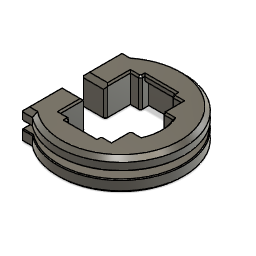
PSUThing (Autodesk Fusion 360 design; units mm, degrees)
Autodesk Fusion 360 part; units mm, degrees
sketch "Skizze1" plane through (0, 0, 0) normal (0, 1, 0) x (1, 0, 0)
  circle A0 centre (0, 0) radius 12.1
  circle A1 centre (0, 0) radius 10.1
  line L0 (0, 0) -> (-40.078, 0) construction
  line L1 (-12.5, 9.6) -> (-12.5, -9.6)
  line L2 (0, 0) -> (20.9765, 0) construction
  line L3 (-12.5, 9.6) -> (-7.3655, 9.6)
  line L4 (-12.5, -9.6) -> (-7.3655, -9.6)
  line L5 (6.5, -10) -> (-6.5, -10)
  line L6 (-6.5, -10) -> (-6.5, 10)
  line L7 (-6.5, 10) -> (6.5, 10)
  line L8 (6.5, 10) -> (6.5, -10)
  line L9 (6.5, -10) -> (-6.5, 10) construction
  line L10 (-6.5, -10) -> (6.5, 10) construction
  line L11 (-3.9, -10) -> (-3.9, 10)
  line L12 (3.9, -10) -> (3.9, 10)
  line L13 (-6.5, -8.9) -> (-3.9, -8.9)
  line L14 (-6.5, 8.9) -> (-3.9, 8.9)
  line L15 (3.9, 8.9) -> (6.5, 8.9)
  line L16 (3.9, -8.9) -> (6.5, -8.9)
  line L17 (6.5, -4) -> (9.2742, -4)
  line L18 (6.5, 4) -> (9.2742, 4)
  point P0 (-12.5, 0)
  point P1 (12.1, 0)
  dimension "d2" = 24.2
  dimension "d3" = 2
  dimension "d4" = 24.6
  dimension "d5" = 19.2
  dimension "d6" = 13
  dimension "d7" = 20
  dimension "d10" = 2.6
  dimension "d11" = 2.6
  dimension "d12" = 1.1
  dimension "d13" = 1.1
  dimension "d14" = 1.1
  dimension "d15" = 1.1
  dimension "d16" = 4
  constraint coincident A0.centre A1.centre
  constraint horizontal L0
  constraint perpendicular L0 L1
  constraint midpoint L1 P0
  constraint coincident L0 P0
  constraint parallel L0 L2
  constraint coincident L2 P1
  constraint coincident A0 P1
  constraint coincident A0 L3.end
  constraint perpendicular L1 L3
  constraint coincident A0 L4.end
  constraint perpendicular L1 L4
  constraint horizontal L5
  constraint perpendicular L5 L6
  constraint parallel L5 L7
  constraint parallel L6 L8
  constraint coincident L9 A0.centre
  constraint coincident L10 A0.centre
  constraint coincident L2 A0.centre
  constraint coincident L5 L11.start
  constraint coincident L7 L11.end
  constraint perpendicular L7 L11
  constraint coincident L5 L12.start
  constraint coincident L7 L12.end
  constraint perpendicular L7 L12
  constraint coincident L6 L13.start
  constraint coincident L11 L13.end
  constraint perpendicular L11 L13
  constraint coincident L6 L14.start
  constraint coincident L11 L14.end
  constraint perpendicular L11 L14
  constraint coincident L12 L15.start
  constraint coincident L8 L15.end
  constraint perpendicular L8 L15
  constraint coincident L12 L16.start
  constraint coincident L8 L16.end
  constraint perpendicular L8 L16
  constraint coincident L8 L17.start
  constraint coincident A1 L17.end
  constraint perpendicular L8 L17
  constraint symmetric L2 L17.start L18.start
  constraint symmetric L2 L17.end L18.end
  measures "d2" diameter of A0
  measures "d3" distance of A0 A1
  measures "d4" distance of P0 P1
  measures "d6" distance of L6.end L7.end
  measures "d7" distance of L5.end L6.end
  measures "d10" distance of L8 L12
  measures "d11" distance of L6 L11
  measures "d12" distance of L5 L16
  measures "d13" distance of L5 L13
  measures "d14" distance of L7 L14
  measures "d15" distance of L7 L15
  measures "d16" distance of L2 L17
extrude "Extrusion1" add sketch "Skizze1" along normal mid plane 1.8 contours A0 | A0 L1 L3 L4 | A1 L8 L18 | A1 L8 L17 | A1 L12 L15 | A1 L7 L8 L12 L15 | A1 L5 L8 L12 L16 | A1 L12 L16 | A1 L7 | A1 L5 | A1 L11 L14 | A1 L6 L7 L11 L14 | A1 L5 L6 L11 L13 | A1 L11 L13 | A1 L6 makes body 1
sketch "Skizze2" plane through (0, -0.9, 0) normal (0, -1, 0) x (1, 0, 0)
  line L0 (3.9, -8.9) -> (3.9, -10)
  line L1 (3.9, -10) -> (-3.9, -10)
  line L2 (-3.9, -10) -> (-3.9, -8.9)
  line L3 (-3.9, -8.9) -> (-6.5, -8.9)
  line L4 (-6.5, -8.9) -> (-6.5, 8.9)
  line L5 (-6.5, 8.9) -> (-3.9, 8.9)
  line L6 (-3.9, 8.9) -> (-3.9, 10)
  line L7 (-3.9, 10) -> (3.9, 10)
  line L8 (3.9, 10) -> (3.9, 8.9)
  line L9 (3.9, 8.9) -> (6.5, 8.9)
  line L10 (6.5, 8.9) -> (6.5, 4)
  line L11 (6.5, 4) -> (9.2742, 4)
  arc A0 (9.2742, -4) -> (9.2742, 4) centre (0, 0) ccw
  line L12 (9.2742, -4) -> (6.5, -4)
  line L13 (6.5, -4) -> (6.5, -8.9)
  line L14 (6.5, -8.9) -> (3.9, -8.9)
  line L15 (-12.5, 9.6) -> (-12.5, -9.6)
  line L16 (-12.5, -9.6) -> (-7.3655, -9.6)
  arc A1 (-7.3655, -9.6) -> (-7.3655, 9.6) centre (0, 0) ccw
  line L17 (-7.3655, 9.6) -> (-12.5, 9.6)
  arc A2 (-9.8003, -12.7736) -> (-9.8003, 12.7736) centre (0, 0) ccw
  line L18 (-12.5, 9.6) -> (-12.5, 17.8119) construction
  line L19 (-12.5, -9.6) -> (-12.5, -17.8838) construction
  line L20 (-9.8003, 12.7736) -> (-12.5, 12.7736)
  line L21 (-12.5, 9.6) -> (-12.5, 12.7736)
  line L22 (-9.8003, -12.7736) -> (-12.5, -12.7736)
  line L23 (-12.5, -12.7736) -> (-12.5, -9.6)
  dimension "d18" = 4
  constraint coincident L15.start L17.end
  constraint perpendicular L17 L18
  constraint coincident L15.end L16.start
  constraint perpendicular L16 L19
  constraint coincident L18 L20.end
  constraint perpendicular L18 L20
  constraint coincident L19 L22.end
  constraint perpendicular L19 L22
extrude "Extrusion2" add sketch "Skizze2" along normal blind 3 bodies 1
sketch "Skizze3" plane through (0, 0.9, 0) normal (0, 1, 0) x (-1, 0, 0)
  line L0 (-3.9, -10) -> (-3.9, -8.9)
  line L1 (-3.9, -8.9) -> (-6.5, -8.9)
  line L2 (-6.5, -8.9) -> (-6.5, -4)
  line L3 (-6.5, -4) -> (-9.2742, -4)
  arc A0 (-9.2742, 4) -> (-9.2742, -4) centre (0, 0) ccw
  line L4 (-9.2742, 4) -> (-6.5, 4)
  line L5 (-6.5, 4) -> (-6.5, 8.9)
  line L6 (-6.5, 8.9) -> (-3.9, 8.9)
  line L7 (-3.9, 8.9) -> (-3.9, 10)
  line L8 (-3.9, 10) -> (3.9, 10)
  line L9 (3.9, 10) -> (3.9, 8.9)
  line L10 (3.9, 8.9) -> (6.5, 8.9)
  line L11 (6.5, 8.9) -> (6.5, -8.9)
  line L12 (6.5, -8.9) -> (3.9, -8.9)
  line L13 (3.9, -8.9) -> (3.9, -10)
  line L14 (3.9, -10) -> (-3.9, -10)
  line L15 (12.5, -9.6) -> (12.5, 9.6)
  line L16 (12.5, 9.6) -> (7.3655, 9.6)
  arc A1 (7.3655, 9.6) -> (7.3655, -9.6) centre (0, 0) ccw
  line L17 (7.3655, -9.6) -> (12.5, -9.6)
  line L18 (12.5, -12.7736) -> (12.5, -9.6)
  line L19 (9.8003, -12.7736) -> (12.5, -12.7736)
  arc A2 (9.8003, 12.7736) -> (9.8003, -12.7736) centre (0, 0) ccw
  line L20 (9.8003, 12.7736) -> (12.5, 12.7736)
  line L21 (12.5, 9.6) -> (12.5, 12.7736)
extrude "Extrusion3" add sketch "Skizze3" along normal blind 3 bodies 1
sketch "Skizze4" plane through (0, 3.9, 0) normal (0, 1, 0) x (-1, 0, 0)
  arc A0 (-9.2742, 4) -> (-9.2742, -4) centre (0, 0) ccw
  line L0 (-9.2742, 4) -> (-6.5, 4)
  line L1 (-6.5, 4) -> (-6.5, 8.9)
  line L2 (-6.5, 8.9) -> (-3.9, 8.9)
  line L3 (-3.9, 8.9) -> (-3.9, 10)
  line L4 (-3.9, 10) -> (3.9, 10)
  line L5 (3.9, 10) -> (3.9, 8.9)
  line L6 (3.9, 8.9) -> (6.5, 8.9)
  line L7 (6.5, 8.9) -> (6.5, -8.9)
  line L8 (6.5, -8.9) -> (3.9, -8.9)
  line L9 (3.9, -8.9) -> (3.9, -10)
  line L10 (3.9, -10) -> (-3.9, -10)
  line L11 (-3.9, -10) -> (-3.9, -8.9)
  line L12 (-3.9, -8.9) -> (-6.5, -8.9)
  line L13 (-6.5, -8.9) -> (-6.5, -4)
  line L14 (-6.5, -4) -> (-9.2742, -4)
  arc A1 (9.8003, 12.7736) -> (9.8003, -12.7736) centre (0, 0) ccw
  line L15 (9.8003, -12.7736) -> (12.5, -12.7736)
  line L16 (12.5, -12.7736) -> (12.5, 12.7736)
  line L17 (12.5, 12.7736) -> (9.8003, 12.7736)
  line L18 (0, 0) -> (25.167, 0) construction
  line L19 (6.5, 0) -> (12.5, 0) construction
  line L20 (6.5, 2.5) -> (12.5, 2.5)
  line L21 (12.5, 2.5) -> (12.5, -2.5)
  line L22 (12.5, -2.5) -> (6.5, -2.5)
  line L23 (6.5, -2.5) -> (6.5, 2.5)
  line L24 (6.5, 2.5) -> (12.5, -2.5) construction
  line L25 (12.5, 2.5) -> (6.5, -2.5) construction
  point P0 (9.5, 0)
  point P1 (9.5, 0)
  dimension "d25" = 5
  constraint coincident A0.centre A1.centre
  constraint perpendicular L16 L18
  constraint midpoint L7 L19.start
  constraint midpoint L16 L19.end
  constraint midpoint L19 P1
  constraint horizontal L20
  constraint perpendicular L20 L21
  constraint parallel L20 L22
  constraint parallel L21 L23
  constraint coincident L7 L20.start
  constraint coincident L24 P1
  constraint coincident L25 P1
  constraint coincident P1 P0
  measures "d25" distance of L20 L22
extrude "Extrusion4" cut sketch "Skizze4" against normal up to surface (7.8 mm away) contours L7 L16 L20 L21 L22 L23 bodies 1
sketch "Skizze5" plane through (0, -3.9, 0) normal (0, -1, 0) x (1, 0, 0)
  line L0 (-6.5, -2.5) -> (-12.5, -2.5)
  line L1 (-12.5, -2.5) -> (-12.5, -12.7736)
  line L2 (-12.5, -12.7736) -> (-9.8003, -12.7736)
  arc A0 (-9.8003, -12.7736) -> (-9.8003, 12.7736) centre (0, 0) ccw
  line L3 (-9.8003, 12.7736) -> (-12.5, 12.7736)
  line L4 (-12.5, 12.7736) -> (-12.5, 2.5)
  line L5 (-12.5, 2.5) -> (-6.5, 2.5)
  line L6 (-6.5, 2.5) -> (-6.5, 8.9)
  line L7 (-6.5, 8.9) -> (-3.9, 8.9)
  line L8 (-3.9, 8.9) -> (-3.9, 10)
  line L9 (-3.9, 10) -> (3.9, 10)
  line L10 (3.9, 10) -> (3.9, 8.9)
  line L11 (3.9, 8.9) -> (6.5, 8.9)
  line L12 (6.5, 8.9) -> (6.5, 4)
  line L13 (6.5, 4) -> (9.2742, 4)
  arc A1 (9.2742, -4) -> (9.2742, 4) centre (0, 0) ccw
  line L14 (9.2742, -4) -> (6.5, -4)
  line L15 (6.5, -4) -> (6.5, -8.9)
  line L16 (6.5, -8.9) -> (3.9, -8.9)
  line L17 (3.9, -8.9) -> (3.9, -10)
  line L18 (3.9, -10) -> (-3.9, -10)
  line L19 (-3.9, -10) -> (-3.9, -8.9)
  line L20 (-3.9, -8.9) -> (-6.5, -8.9)
  line L21 (-6.5, -8.9) -> (-6.5, -2.5)
  line L22 (-3.9, 10) -> (3.9, 10)
  line L23 (3.9, 10) -> (3.9, 11)
  line L24 (3.9, 11) -> (-3.9, 11)
  line L25 (-3.9, 11) -> (-3.9, 10)
  line L26 (0, 0) -> (-17.587, 0) construction
  line L27 (3.9, -11) -> (-3.9, -11)
  line L28 (-3.9, -11) -> (-3.9, -10)
  line L29 (3.9, -10) -> (3.9, -11)
  line L30 (-3.9, -10) -> (3.9, -10)
  dimension "d28" = 1
  constraint perpendicular L22 L23
  constraint parallel L22 L24
  constraint parallel L23 L25
  constraint coincident L9.end L10.start
  constraint perpendicular L10 L22
  constraint coincident L8.end L9.start
  constraint coincident A0.centre A1.centre
  constraint horizontal L26
  constraint symmetric L8.end L26 L18.end
  constraint symmetric L9.end L26 L17.end
  constraint symmetric L23.end L26 L27.start
  constraint symmetric L24.end L26 L27.end
  measures "d28" distance of L8.end L24.end
extrude "Extrusion5" cut sketch "Skizze5" against normal up to surface (6.2 mm away) contours L18 L27 L28 L29 L30 | L9 L22 L23 L24 L25 bodies 1
chamfer "Fase1" distance 1 angle 45 7 edges at (-12.5, 3.9, -7.6368) (-9.5, 3.9, -2.5) (-9.5, 3.9, 2.5) (-12.5, 3.9, 7.6368) (-11.1502, 3.9, 12.7736) (16.1, 3.9, 0) (-11.1502, 3.9, -12.7736) on bodies 1
chamfer "Fase2" distance 0.5 angle 45 8 edges at (-6.5, -0.5, -2.5) (-3.9, 0, -8.9) (3.9, 0, -8.9) (6.5, 0, -4) (6.5, 0, 4) (3.9, 0, 8.9) (-3.9, 0, 8.9) (-6.5, -0.5, 2.5) on bodies 1
chamfer "Fase3" distance 0.2 angle 45 2 edges at (0, 2.3, 10) (0, 2.3, -10) on bodies 1
chamfer "Fase4" distance 0.4 angle 45 23 edges at (-6.5, 3.9, -6.2) (-5.45, 3.9, -8.9) (-4.15, 3.9, -9.15) (-3.9, 3.9, -9.7) (0, 3.9, -10) (3.9, 3.9, -9.7) (4.15, 3.9, -9.15) (5.45, 3.9, -8.9) (6.5, 3.9, -6.7) (6.75, 3.9, -4.25) (8.1371, 3.9, -4) (10.1, 3.9, 0) (8.1371, 3.9, 4) (6.75, 3.9, 4.25) (6.5, 3.9, 6.7) (5.45, 3.9, 8.9) (4.15, 3.9, 9.15) (3.9, 3.9, 9.7) (0, 3.9, 10) (-3.9, 3.9, 9.7) (-4.15, 3.9, 9.15) (-5.45, 3.9, 8.9) (-6.5, 3.9, 6.2) on bodies 1
chamfer "Fase5" distance 0.5 angle 45 32 edges at (16.1, -3.9, 0) (-11.1502, -3.9, 12.7736) (-12.5, -3.9, 7.6368) (-12.5, -3.9, -7.6368) (-11.1502, -3.9, -12.7736) (-9.75, -3.9, -2.5) (-9.75, -3.9, 2.5) (-6.75, -3.9, 2.75) (-6.5, -3.9, 5.95) (-5.45, -3.9, 8.9) (-4.15, -3.9, 9.15) (-3.9, -3.9, 10.2) (0, -3.9, 11) (3.9, -3.9, 10.2) (4.15, -3.9, 9.15) (5.45, -3.9, 8.9) (6.5, -3.9, 6.7) (6.75, -3.9, 4.25) (8.1371, -3.9, 4) (10.1, -3.9, 0) (8.1371, -3.9, -4) (6.75, -3.9, -4.25) (6.5, -3.9, -6.7) (5.45, -3.9, -8.9) (4.15, -3.9, -9.15) (3.9, -3.9, -10.2) (0, -3.9, -11) (-3.9, -3.9, -10.2) (-4.15, -3.9, -9.15) (-5.45, -3.9, -8.9) (-6.5, -3.9, -5.95) (-6.75, -3.9, -2.75) on bodies 1
chamfer "Fase6" distance 0.2 angle 45 4 edges at (-12.5, -2.15, -12.7736) (-12.5, 1.9, -12.7736) (-12.5, -2.15, 12.7736) (-12.5, 1.9, 12.7736) on bodies 1
chamfer "Fase7" distance 0.2 angle 45 16 edges at (-12.5, 0, -9.6) (-12.5, -0.9, -11.0868) (-12.4, -0.9, -12.6736) (-11.0502, -0.9, -12.7736) (16.1, -0.9, 0) (-12.5, 0.9, -11.0868) (-12.4, 0.9, -12.6736) (-11.0502, 0.9, -12.7736) (16.1, 0.9, 0) (-11.0502, -0.9, 12.7736) (-11.0502, 0.9, 12.7736) (-12.4, 0.9, 12.6736) (-12.5, 0.9, 11.0868) (-12.4, -0.9, 12.6736) (-12.5, -0.9, 11.0868) (-12.5, 0, 9.6) on bodies 1
chamfer "Fase8" distance 0.5 angle 45 2 edges at (-12.5, -0.25, 2.5) (-12.5, -0.25, -2.5) on bodies 1
copy_body "Körper->Berechn1" bodies 1 removing the originals makes body 2 in component "Component"
component "Component" placed x (1, 0, 0) y (0, 1, 0) z (0, 0, 1) at (0, 0, 0)
equation "clearance = 0.4 mm"
equation "d2 = 25 mm - 2 * clearance"
equation "d4 = 25 mm - clearance"
equation "d5 = 20 mm - clearance * 2"
equation "d10 = 3 mm - clearance"
equation "d11 = 3 mm - clearance"
equation "d12 = 1.5 mm - clearance"
equation "d13 = 1.5 mm - clearance"
equation "d14 = 1.5 mm - clearance"
equation "d15 = 1.5 mm - clearance"
equation "Overlap = 4 mm"
equation "d18 = Overlap"
equation "wall_thickness = 3 mm"
equation "d20 = wall_thickness"
equation "d22 = wall_thickness"
equation "slot_width = 5 mm"
equation "d25 = slot_width"
equation "d29 = -2.00 mm + clearance"
